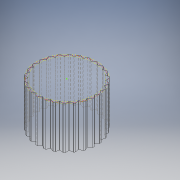
# Autodesk Inventor part: 146842_1
Saved by Autodesk Inventor 2018 (Build 220112000, 112)
## iProperties
Created: 2015-01-24
Part Number: 146842_1
Material: Acciaio, Non legato
Document SubType Name: Modeling
Designer: Manuel
Density: 7.85 g/cm^3
Appearance: Acciaio
Mass: 93.7385 g
Surface Area: 34.4559 cm^2
Volume: 11.9412 cm^3
Author: LUT
Autodesk Inventor part; units mm, degrees
ref_plane "YZ Plane" through (0, 0, 0) normal (1, 0, 0) x (0, 1, 0)
ref_plane "XZ Plane" through (0, 0, 0) normal (0, 1, 0) x (-1, 0, 0)
ref_plane "XY Plane" through (0, 0, 0) normal (0, 0, 1) x (1, 0, 0)
sketch "Schizzo1" plane through (0, 0, 0) normal (0, 0, 1) x (1, 0, 0)
  spline S0 degree 4 poles (0.4173, 14.2471) (0.8843, 13.781) (1.4764, 13.0957) (2.0648, 12.1644) (2.592, 10.8862) (2.7089, 10.1519) (2.7777, 9.6413) (2.6932, 9.3481) knots 0 0 0 0 0 0.436491 0.603339 0.764764 1 1 1 1 1
  arc A0 (0.3921, 14.2479) -> (-0.3921, 14.2479) centre (0, 0) ccw
  line L0 (0, 0) -> (0, 14.2532) construction
  spline S1 degree 4 poles (-0.4173, 14.2471) (-0.8843, 13.781) (-1.4764, 13.0957) (-2.0648, 12.1644) (-2.592, 10.8862) (-2.7089, 10.1519) (-2.7777, 9.6413) (-2.6932, 9.3481) knots 0 0 0 0 0 0.436491 0.603339 0.764764 1 1 1 1 1
  line L1 (0, 14.2532) -> (0, 0) construction
  line L2 (-2.6932, 9.3481) -> (2.6932, 9.3481) construction
  line L3 (-2.6932, 9.3481) -> (0, 0)
  line L4 (0, 0) -> (2.6932, 9.3481)
  line L5 (-1.2527, 4.3481) -> (1.2527, 4.3481)
  arc A1 (-0.3921, 14.2479) -> (-0.4352, 14.2293) centre (-0.3904, 14.1846) ccw
  arc A2 (0.4352, 14.2293) -> (0.3921, 14.2479) centre (0.3904, 14.1846) ccw
  point P0 (1.1398, 13.4509)
  point P1 (1.7346, 12.6263)
  point P2 (2.1979, 11.7876)
  point P3 (2.5243, 10.9494)
  point P4 (2.7033, 10.1279)
  point P5 (-1.1398, 13.4509)
  point P6 (-1.7346, 12.6263)
  point P7 (-2.1979, 11.7876)
  point P8 (-2.5243, 10.9494)
  point P9 (-2.7033, 10.1279)
  point P10 (-0.4352, 14.2293)
  point P11 (-0.4352, 14.2293)
  point P12 (0.4352, 14.2293)
  point P13 (0.4352, 14.2293)
  dimension "d0" = 14.2471
  dimension "d1" = 0.4173
  dimension "d2" = 13.4509
  dimension "d3" = 1.1398
  dimension "d4" = 12.6263
  dimension "d5" = 1.7346
  dimension "d6" = 11.7876
  dimension "d7" = 2.1979
  dimension "d8" = 10.9494
  dimension "d9" = 2.5243
  dimension "d10" = 10.1279
  dimension "d11" = 2.7033
  dimension "d12" = 9.3481
  dimension "d13" = 2.6932
  dimension "d50" = 5
  dimension "d276" = 0.1266
  dimension "d277" = 0.1266
  dimension "d279" = 0
  dimension "d280" = 0
  constraints: 12 end point, 11 point on circle, 7 symmetric about line, 3 centre point, 2 coincident, 2 point on line, 2 tangent, 1 collinear, 1 horizontal, 1 perpendicular, 1 vertical, 24 other
  measures "d0" vertical distance of point (0.417, 14.247) point (0, 0)
  measures "d1" horizontal distance of point (0.417, 14.247) point (0, 0)
  measures "d2" vertical distance of point (1.14, 13.451) point (0, 0)
  measures "d3" horizontal distance of point (1.14, 13.451) point (0, 0)
  measures "d4" vertical distance of point (1.735, 12.626) point (0, 0)
  measures "d5" horizontal distance of point (1.735, 12.626) point (0, 0)
  measures "d6" vertical distance of point (2.198, 11.788) point (0, 0)
  measures "d7" horizontal distance of point (2.198, 11.788) point (0, 0)
  measures "d8" vertical distance of point (2.524, 10.949) point (0, 0)
  measures "d9" horizontal distance of point (2.524, 10.949) point (0, 0)
  measures "d10" vertical distance of point (2.703, 10.128) point (0, 0)
  measures "d11" horizontal distance of point (2.703, 10.128) point (0, 0)
  measures "d12" vertical distance of L2.end point (0, 0)
  measures "d13" horizontal distance of L2.end point (0, 0)
  measures "d50" distance between parallel lines of L5 L2
  measures "d276" diameter of A1
  measures "d277" diameter of A2
  measures "d279" distance of point (-0.435, 14.229) point (-0.435, 14.229)
  measures "d280" distance of point (0.435, 14.229) point (0.435, 14.229)
extrude "Estrusione28" add sketch "Schizzo1" along normal blind 20 contours S0 L4 L5 L3 S1 A1 A0 A2
pattern_circular "Serie circolare9" count 26 over 360 about axis through (0, 0, -10) along (0, 0, 1)
sketch "Schizzo40" plane through (0, 0, 0) normal (0, 0, -1) x (-1, 0, 0)
  circle A0 centre (0, 0) radius 13.055
  circle A1 centre (0, 0) radius 13.7866 construction
  circle A2 centre (0, 0) radius 14.2532 construction
  dimension "d286" = 26.11
  dimension "d319" = 27.5733
  dimension "d320" = 28.5065
  constraints: 3 centre point, 3 coincident
  measures "d286" diameter of A0
  measures "d319" diameter of A1
  measures "d320" diameter of A2
extrude "Estrusione29 diametro fondo" add sketch "Schizzo40" against normal blind 20
sketch "Schizzo41" plane through (0, 0, 20) normal (0, 0, 1) x (1, 0, 0)
  circle A0 centre (0, 0) radius 13.055 construction
  circle A1 centre (0, 0) radius 13.7866 construction
  circle A2 centre (0, 0) radius 14.2532
  circle A3 centre (0, 0) radius 13.055 construction
  circle A4 centre (0, 0) radius 13.7866 construction
  circle A5 centre (0, 0) radius 14.2532 construction
  circle A6 centre (0, 0) radius 13.055 construction
  circle A7 centre (0, 0) radius 13.7866 construction
  circle A8 centre (0, 0) radius 14.2532 construction
  circle A9 centre (0, 0) radius 13.055 construction
  circle A10 centre (0, 0) radius 13.7866 construction
  circle A11 centre (0, 0) radius 14.2532 construction
  circle A12 centre (0, 0) radius 28.0399
  dimension "d289" = 27.5733
  dimension "d_interno_attuale" = 26.11
  dimension "d291" = 28.5065
  dimension "d292" = 27.5733
  dimension "d293" = 26.11
  dimension "d294" = 28.5065
  dimension "d301" = 27.5733
  dimension "d302" = 26.11
  dimension "d303" = 28.5065
  dimension "d304" = 27.5733
  dimension "d305" = 26.11
  dimension "d306" = 28.5065
  dimension "d321" = 56.0798
  constraints: 13 centre point, 13 coincident
  measures "d289" diameter of A1
  measures "d_interno_attuale" diameter of A0
  measures "d291" diameter of A2
  measures "d292" diameter of A4
  measures "d293" diameter of A3
  measures "d294" diameter of A5
  measures "d301" diameter of A7
  measures "d302" diameter of A6
  measures "d303" diameter of A8
  measures "d304" diameter of A10
  measures "d305" diameter of A9
  measures "d306" diameter of A11
  measures "d321" diameter of A12
extrude "Estrusione30" cut sketch "Schizzo41" against normal blind 20
sketch "Schizzo42" plane through (0, 0, 20) normal (0, 0, 1) x (1, 0, 0)
  circle A0 centre (0, 0) radius 13.055 construction
  circle A1 centre (0, 0) radius 14.2532 construction
  circle A2 centre (0, 0) radius 13.7866 construction
  dimension "d324" = 27.5733
  dimension "d325" = 28.5065
  dimension "d326" = 26.11
  constraints: 3 centre point, 3 coincident
  measures "d324" diameter of A2
  measures "d325" diameter of A1
  measures "d326" diameter of A0
equation "\"d0\" = y1"
equation "\"d1\" = x1"
equation "\"d2\" = y2"
equation "\"d3\" = x2"
equation "\"d4\" = y3"
equation "\"d5\" = x3"
equation "\"d6\" = y4"
equation "\"d7\" = x4"
equation "\"d8\" = y5"
equation "\"d9\" = x5"
equation "\"d10\" = y6"
equation "\"d11\" = x6"
equation "\"d12\" = y7"
equation "\"d13\" = x7"
equation "\"x7\" = 2.69324"
equation "\"x4\" = 2.19787"
equation "\"y2\" = 13.45088"
equation "\"x1\" = 0.41734"
equation "\"y1\" = 14.24714"
equation "\"x5\" = 2.52434"
equation "\"x6\" = 2.70329"
equation "\"y6\" = 10.12789"
equation "\"y7\" = 9.34807"
equation "\"y5\" = 10.9494"
equation "\"x3\" = 1.73461"
equation "\"x2\" = 1.13983"
equation "\"y3\" = 12.62634"
equation "\"y4\" = 11.78763"
equation "\"pel2\" = 621.98261"
equation "\"pel1\" = 460.56452"
equation "\"D_prerullatura\" = 27.57327"
equation "\"D_Interno_finito\" = 26.11"
equation "\"D_Esterno_finito\" = 28.5065"
equation "\"D_Interno_maggiorazione\" = -1.46327"
equation "\"D_Esterno_maggiorazione\" = 0.93323"
equation "\"d295\" = 27.57327"
equation "\"d296\" = -1.46327"
equation "\"d297\" = 0.93323"
equation "\"d299\" = 26.11"
equation "\"d300\" = 28.5065"
equation "\"d307\" = 27.57327"
equation "\"d308\" = 27.57327"
equation "\"d309\" = -1.46327"
equation "\"d310\" = 0.93323"
equation "\"d311\" = -1.46327"
equation "\"d312\" = 0.93323"
equation "\"d315\" = 26.11"
equation "\"d316\" = 28.5065"
equation "\"d317\" = 26.11"
equation "\"d318\" = 28.5065"
equation "\"d327\" = 27.57327"
equation "\"d328\" = 28.5065"
equation "\"d329\" = 26.11"
